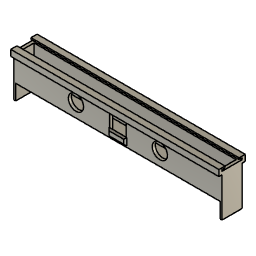
Magic Mirror Case (Autodesk Fusion 360 design; units mm, degrees)
part number: 2025-08-01-03-08-55-904
Autodesk Fusion 360 part; units mm, degrees
sketch "Sketch1" plane through (0, 0, 0) normal (0, 1, 0) x (1, 0, 0)
  line L0 (-63.2319, -37.0078) -> (276.7681, -37.0078)
  line L1 (276.7681, -37.0078) -> (276.7681, 6.9922)
  line L2 (276.7681, 6.9922) -> (-63.2319, 6.9922)
  line L3 (-63.2319, 6.9922) -> (-63.2319, -37.0078)
  line L4 (93.2681, -35.0078) -> (120.2681, -35.0078)
  line L5 (120.2681, -35.0078) -> (120.2681, 4.9922)
  line L6 (120.2681, 4.9922) -> (93.2681, 4.9922)
  line L7 (93.2681, 4.9922) -> (93.2681, -35.0078)
  dimension "d1" = 340
  dimension "d2" = 44
  dimension "d3" = 27
  dimension "d4" = 40
  dimension "d5" = 156.5
  dimension "d6" = 2
  constraint horizontal L0
  constraint vertical L1
  constraint horizontal L2
  constraint vertical L3
  constraint horizontal L4
  constraint vertical L5
  constraint horizontal L6
  constraint vertical L7
  measures "d1" distance of L0.start L0.end
  measures "d2" distance of L0.start L2.end
  measures "d3" distance of L4.start L4.end
  measures "d4" distance of L4.start L6.end
  measures "d5" distance of L3 L7
  measures "d6" distance of L0 L4
extrude "Extrude1" add sketch "Sketch1" along normal blind 5 makes body 1
sketch "Sketch2" plane through (0, 0, 0) normal (0, -1, 0) x (1, 0, 0)
  line L0 (93.2681, -4.9922) -> (93.2681, 35.0078)
  line L1 (93.2681, 35.0078) -> (120.2681, 35.0078)
  line L2 (120.2681, 35.0078) -> (120.2681, -4.9922)
  line L3 (120.2681, -4.9922) -> (93.2681, -4.9922)
  line L4 (-63.2319, 37.0078) -> (-63.2319, -6.9922)
  line L5 (-63.2319, -6.9922) -> (276.7681, -6.9922)
  line L6 (276.7681, -6.9922) -> (276.7681, 37.0078)
  line L7 (276.7681, 37.0078) -> (-63.2319, 37.0078)
  line L8 (92.2681, -4.9922) -> (121.2681, -4.9922)
  line L9 (121.2681, -4.9922) -> (121.2681, 7.0078)
  line L10 (121.2681, 7.0078) -> (92.2681, 7.0078)
  line L11 (92.2681, 7.0078) -> (92.2681, -4.9922)
  dimension "d9" = 29
  dimension "d10" = 12
  dimension "d11" = 2
  dimension "d12" = 155.5
  constraint horizontal L8
  constraint vertical L9
  constraint horizontal L10
  constraint vertical L11
  measures "d9" distance of L8.start L8.end
  measures "d10" distance of L8.start L10.end
  measures "d11" distance of L5 L8
  measures "d12" distance of L4 L11
extrude "Extrude2" add sketch "Sketch2" along normal blind 2.5 draft -45 separate body contours L0 L8 L10 L11 | L0 L2 L3 L8 L10 | L2 L8 L9 L10 makes body 2
sketch "Sketch3" plane through (0, 5, 0) normal (0, 1, 0) x (-1, 0, 0)
  line L0 (-93.2681, 35.0078) -> (-93.2681, -4.9922)
  line L1 (-93.2681, -4.9922) -> (-120.2681, -4.9922)
  line L2 (-120.2681, -4.9922) -> (-120.2681, 35.0078)
  line L3 (-120.2681, 35.0078) -> (-93.2681, 35.0078)
  line L4 (63.2319, -6.9922) -> (63.2319, 37.0078)
  line L5 (63.2319, 37.0078) -> (-276.7681, 37.0078)
  line L6 (-276.7681, 37.0078) -> (-276.7681, -6.9922)
  line L7 (-276.7681, -6.9922) -> (63.2319, -6.9922)
  line L8 (-276.7681, -6.9922) -> (63.2319, -6.9922)
  line L9 (63.2319, -6.9922) -> (63.2319, -4.9922)
  line L10 (63.2319, -4.9922) -> (-276.7681, -4.9922)
  line L11 (-276.7681, -4.9922) -> (-276.7681, -6.9922)
  line L12 (-276.7681, 37.0078) -> (-271.7681, 37.0078)
  line L13 (-271.7681, 37.0078) -> (-271.7681, -4.9922)
  line L14 (-271.7681, -4.9922) -> (-276.7681, -4.9922)
  line L15 (-276.7681, -4.9922) -> (-276.7681, 37.0078)
  line L16 (63.2319, 37.0078) -> (58.2319, 37.0078)
  line L17 (58.2319, 37.0078) -> (58.2319, -4.9922)
  line L18 (58.2319, -4.9922) -> (63.2319, -4.9922)
  line L19 (63.2319, -4.9922) -> (63.2319, 37.0078)
  dimension "d15" = 2
  dimension "d16" = 5
  dimension "d17" = 5
  constraint horizontal L8
  constraint vertical L9
  constraint horizontal L10
  constraint vertical L11
  constraint coincident L6.end L7.start
  constraint horizontal L12
  constraint vertical L13
  constraint horizontal L14
  constraint vertical L15
  constraint coincident L5.end L6.start
  constraint horizontal L16
  constraint vertical L17
  constraint horizontal L18
  constraint vertical L19
  constraint coincident L4.end L5.start
  measures "d15" distance of L6.end L10.end
  measures "d16" distance of L5.end L12.end
  measures "d17" distance of L4.end L16.end
extrude "Extrude3" add sketch "Sketch3" along normal blind 28 contours L1 L4 L6 L7 L8 L9 L10 L11 L14 L18 | L4 L5 L10 L16 L17 L18 L19 | L5 L6 L10 L12 L13 L14 L15 bodies 1
sketch "Sketch4" plane through (0, 0, -4.9922) normal (0, 0, 1) x (-1, 0, 0)
  line L0 (-93.2681, 0) -> (-120.2681, 0)
  line L1 (-120.2681, 0) -> (-120.2681, -5)
  line L2 (-120.2681, -5) -> (-271.7681, -5)
  line L3 (-271.7681, -5) -> (-271.7681, -33)
  line L4 (-271.7681, -33) -> (58.2319, -33)
  line L5 (58.2319, -33) -> (58.2319, -5)
  line L6 (58.2319, -5) -> (-93.2681, -5)
  line L7 (-93.2681, -5) -> (-93.2681, 0)
  line L8 (-271.7681, -33) -> (58.2319, -33)
  line L9 (58.2319, -33) -> (58.2319, -28)
  line L10 (58.2319, -28) -> (-271.7681, -28)
  line L11 (-271.7681, -28) -> (-271.7681, -33)
  dimension "d20" = 5
  constraint horizontal L8
  constraint vertical L9
  constraint horizontal L10
  constraint vertical L11
  constraint coincident L5 L9.end
  constraint coincident L3.end L4.start
  measures "d20" distance of L3.end L10.end
extrude "Extrude4" add sketch "Sketch4" along normal blind 42 contours L3 L4 L5 L8 L9 L10 L11 bodies 1
sketch "Sketch5" plane through (0, 0, 0) normal (0, -1, 0) x (1, 0, 0)
  line L0 (93.2681, -4.9922) -> (93.2681, 35.0078)
  line L1 (93.2681, 35.0078) -> (120.2681, 35.0078)
  line L2 (120.2681, 35.0078) -> (120.2681, -4.9922)
  line L3 (120.2681, -4.9922) -> (93.2681, -4.9922)
  line L4 (-63.2319, 37.0078) -> (-63.2319, -6.9922)
  line L5 (-63.2319, -6.9922) -> (276.7681, -6.9922)
  line L6 (276.7681, -6.9922) -> (276.7681, 37.0078)
  line L7 (276.7681, 37.0078) -> (-63.2319, 37.0078)
  circle A0 centre (38.2681, 15.0078) radius 12.5
  circle A1 centre (175.2681, 15.0078) radius 12.5
  dimension "d23" = 25
  dimension "d24" = 22
  dimension "d25" = 55
  dimension "d26" = 25
  dimension "d27" = 22
  dimension "d28" = 55
  measures "d23" diameter of A0
  measures "d24" distance of L5 A0.centre
  measures "d25" distance of L0 A0.centre
  measures "d26" diameter of A1
  measures "d27" distance of L7 A1.centre
  measures "d28" distance of L2 A1.centre
extrude "Extrude5" cut sketch "Sketch5" against normal blind 5 contours A0 | A1 bodies 1
sketch "Sketch6" plane through (0, 33, 0) normal (0, 1, 0) x (-1, 0, 0)
  line L0 (-276.7681, 37.0078) -> (-276.7681, -6.9922)
  line L1 (-276.7681, -6.9922) -> (63.2319, -6.9922)
  line L2 (63.2319, -6.9922) -> (63.2319, 37.0078)
  line L3 (63.2319, 37.0078) -> (-276.7681, 37.0078)
  line L4 (63.2319, 37.0078) -> (-276.7681, 37.0078)
  line L5 (-276.7681, 37.0078) -> (-276.7681, 32.0078)
  line L6 (-276.7681, 32.0078) -> (63.2319, 32.0078)
  line L7 (63.2319, 32.0078) -> (63.2319, 37.0078)
  dimension "d31" = 5
  constraint horizontal L4
  constraint vertical L5
  constraint horizontal L6
  constraint vertical L7
  constraint coincident L2.end L3.start
  measures "d31" distance of L2.end L6.end
extrude "Extrude6" add sketch "Sketch6" along normal blind 5 contours L0 L2 L3 L4 L5 L6 L7 bodies 1
sketch "Sketch7" plane through (0, 0, 37.0078) normal (0, 0, 1) x (-1, 0, 0)
  line L0 (63.2319, -38) -> (63.2319, 0)
  line L1 (63.2319, 0) -> (-276.7681, 0)
  line L2 (-276.7681, 0) -> (-276.7681, -38)
  line L3 (-276.7681, -38) -> (63.2319, -38)
  line L4 (58.2319, -28) -> (-271.7681, -28)
  line L5 (-271.7681, -28) -> (-271.7681, -5)
  line L6 (-271.7681, -5) -> (58.2319, -5)
  line L7 (58.2319, -5) -> (58.2319, -28)
  line L8 (-276.7681, -38) -> (63.2319, -38)
  line L9 (63.2319, -38) -> (63.2319, -33)
  line L10 (63.2319, -33) -> (-276.7681, -33)
  line L11 (-276.7681, -33) -> (-276.7681, -38)
  dimension "d34" = 5
  constraint horizontal L8
  constraint vertical L9
  constraint horizontal L10
  constraint vertical L11
  constraint coincident L2.end L3.start
  measures "d34" distance of L2.end L10.end
extrude "Extrude7" add sketch "Sketch7" along normal blind 5 contours L0 L2 L3 L8 L9 L10 L11 bodies 1
sketch "Sketch8" plane through (0, 33, 0) normal (0, -1, 0) x (1, 0, 0)
  line L0 (-63.2319, 37.0078) -> (276.7681, 37.0078)
  line L1 (276.7681, 37.0078) -> (276.7681, 42.0078)
  line L2 (276.7681, 42.0078) -> (-63.2319, 42.0078)
  line L3 (-63.2319, 42.0078) -> (-63.2319, 37.0078)
  line L4 (276.7681, 42.0078) -> (-63.2319, 42.0078)
  line L5 (-63.2319, 42.0078) -> (-63.2319, 39.5078)
  line L6 (-63.2319, 39.5078) -> (276.7681, 39.5078)
  line L7 (276.7681, 39.5078) -> (276.7681, 42.0078)
  dimension "d37" = 340
  dimension "d38" = 2.5
  constraint horizontal L4
  constraint vertical L5
  constraint horizontal L6
  constraint vertical L7
  constraint coincident L1.end L2.start
  measures "d37" distance of L1.end L2.end
  measures "d38" distance of L1.end L6.end
extrude "Extrude8" add sketch "Sketch8" along normal blind 5 contours L1 L2 L3 L4 L5 L6 L7 bodies 1
sketch "Sketch9" plane through (0, 0, 0) normal (0, -1, 0) x (1, 0, 0)
  circle A0 centre (175.2681, 15.0078) radius 12.5
  circle A1 centre (38.2681, 15.0078) radius 12.5
  line L0 (93.2681, -4.9922) -> (93.2681, 35.0078)
  line L1 (93.2681, 35.0078) -> (120.2681, 35.0078)
  line L2 (120.2681, 35.0078) -> (120.2681, -4.9922)
  line L3 (120.2681, -4.9922) -> (93.2681, -4.9922)
  line L4 (-63.2319, 37.0078) -> (-63.2319, -6.9922)
  line L5 (-63.2319, -6.9922) -> (276.7681, -6.9922)
  line L6 (276.7681, -6.9922) -> (276.7681, 37.0078)
  line L7 (276.7681, 37.0078) -> (-63.2319, 37.0078)
  line L8 (276.7681, 37.0078) -> (-63.2319, 37.0078)
  line L9 (-63.2319, 37.0078) -> (-63.2319, 32.0078)
  line L10 (-63.2319, 32.0078) -> (276.7681, 32.0078)
  line L11 (276.7681, 32.0078) -> (276.7681, 37.0078)
  dimension "d41" = 5
  constraint horizontal L8
  constraint vertical L9
  constraint horizontal L10
  constraint vertical L11
  constraint coincident L6.end L7.start
  measures "d41" distance of L6.end L10.end
extrude "Extrude9" add sketch "Sketch9" along normal blind 5 contours L0 L1 L2 L4 L6 L7 L8 L9 L10 L11 | L0 L1 L2 L10 bodies 1
sketch "Sketch10" plane through (0, 0, 37.0078) normal (0, 0, 1) x (-1, 0, 0)
  line L0 (-276.7681, -33) -> (63.2319, -33)
  line L1 (63.2319, -33) -> (63.2319, 5)
  line L2 (63.2319, 5) -> (-276.7681, 5)
  line L3 (-276.7681, 5) -> (-276.7681, -33)
  line L4 (58.2319, -28) -> (-271.7681, -28)
  line L5 (-271.7681, -28) -> (-271.7681, -5)
  line L6 (-271.7681, -5) -> (58.2319, -5)
  line L7 (58.2319, -5) -> (58.2319, -28)
  line L8 (-276.7681, 5) -> (63.2319, 5)
  line L9 (63.2319, 5) -> (63.2319, 0)
  line L10 (63.2319, 0) -> (-276.7681, 0)
  line L11 (-276.7681, 0) -> (-276.7681, 5)
  dimension "d44" = 5
  constraint horizontal L8
  constraint vertical L9
  constraint horizontal L10
  constraint vertical L11
  constraint coincident L2.end L3.start
  measures "d44" distance of L2.end L10.end
extrude "Extrude10" add sketch "Sketch10" along normal blind 5 contours L1 L2 L3 L8 L9 L10 L11 bodies 1
sketch "Sketch11" plane through (0, 0, 0) normal (0, 1, 0) x (-1, 0, 0)
  line L0 (-276.7681, 37.0078) -> (63.2319, 37.0078)
  line L1 (63.2319, 37.0078) -> (63.2319, 42.0078)
  line L2 (63.2319, 42.0078) -> (-276.7681, 42.0078)
  line L3 (-276.7681, 42.0078) -> (-276.7681, 37.0078)
  line L4 (63.2319, 42.0078) -> (-276.7681, 42.0078)
  line L5 (-276.7681, 42.0078) -> (-276.7681, 39.5078)
  line L6 (-276.7681, 39.5078) -> (63.2319, 39.5078)
  line L7 (63.2319, 39.5078) -> (63.2319, 42.0078)
  dimension "d47" = 2.5
  constraint horizontal L4
  constraint vertical L5
  constraint horizontal L6
  constraint vertical L7
  constraint coincident L1.end L2.start
  measures "d47" distance of L1.end L6.end
extrude "Extrude11" add sketch "Sketch11" along normal blind 5 contours L1 L2 L3 L4 L5 L6 L7 bodies 1
sketch "Sketch12" plane through (0, 0, -6.9922) normal (0, 0, -1) x (1, 0, 0)
  line L0 (276.7681, 0) -> (-63.2319, 0)
  line L1 (-63.2319, 0) -> (-63.2319, -33)
  line L2 (-63.2319, -33) -> (276.7681, -33)
  line L3 (276.7681, -33) -> (276.7681, 0)
  line L4 (-63.2319, -33) -> (-60.2319, -33)
  line L5 (-60.2319, -33) -> (-60.2319, 0)
  line L6 (-60.2319, 0) -> (-63.2319, 0)
  line L7 (-63.2319, 0) -> (-63.2319, -33)
  line L8 (276.7681, -33) -> (273.7681, -33)
  line L9 (273.7681, -33) -> (273.7681, 0)
  line L10 (273.7681, 0) -> (276.7681, 0)
  line L11 (276.7681, 0) -> (276.7681, -33)
  dimension "d50" = 3
  dimension "d51" = 3
  constraint horizontal L4
  constraint vertical L5
  constraint horizontal L6
  constraint vertical L7
  constraint coincident L1.end L2.start
  constraint horizontal L8
  constraint vertical L9
  constraint horizontal L10
  constraint vertical L11
  constraint coincident L2.end L3.start
  measures "d50" distance of L1.end L4.end
  measures "d51" distance of L2.end L8.end
extrude "Extrude12" add sketch "Sketch12" along normal blind 25 contours L0 L2 L3 L8 L9 L10 L11 | L0 L1 L2 L4 L5 L6 L7 bodies 1
sketch "Sketch13" plane through (0, 0, 0) normal (1, 0, 0) x (0, 1, 0)
sketch "Sketch14" plane through (0, 33, 0) normal (0, 1, 0) x (-1, 0, 0)
  line L0 (63.2319, 32.0078) -> (-276.7681, 32.0078)
  line L1 (-276.7681, 32.0078) -> (-276.7681, -31.9922)
  line L2 (-276.7681, -31.9922) -> (-273.7681, -31.9922)
  line L3 (-273.7681, -31.9922) -> (-273.7681, -6.9922)
  line L4 (-273.7681, -6.9922) -> (60.2319, -6.9922)
  line L5 (60.2319, -6.9922) -> (60.2319, -31.9922)
  line L6 (60.2319, -31.9922) -> (63.2319, -31.9922)
  line L7 (63.2319, -31.9922) -> (63.2319, 32.0078)
  line L8 (-276.7681, -31.9922) -> (63.2319, -31.9922)
  line L9 (63.2319, -31.9922) -> (63.2319, -1.9922)
  line L10 (63.2319, -1.9922) -> (-276.7681, -1.9922)
  line L11 (-276.7681, -1.9922) -> (-276.7681, -31.9922)
  dimension "d54" = 30
  constraint horizontal L8
  constraint vertical L9
  constraint horizontal L10
  constraint vertical L11
  constraint coincident L1.end L2.start
  measures "d54" distance of L1.end L10.end
extrude "Extrude13" add sketch "Sketch14" along normal blind 5 draft -22.5 separate body contours L3 L4 L5 L8 makes body 3
